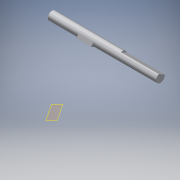
# Autodesk Inventor part: Shaft
Saved by Autodesk Inventor 2017 (Build 210142000, 142)
## iProperties
Created: 2018-02-26
Part Number: Shaft
Material: PAEK Plastic
Document SubType Name: Modeling
Designer: bradl
Density: 1.32 g/cm^3
Appearance: Smooth - White
Author: bradl
Autodesk Inventor part; units mm, degrees
ref_plane "YZ Plane" through (0, 0, 0) normal (1, 0, 0) x (0, 1, 0)
ref_plane "XZ Plane" through (0, 0, 0) normal (0, 1, 0) x (-1, 0, 0)
ref_plane "XY Plane" through (0, 0, 0) normal (0, 0, 1) x (1, 0, 0)
sketch "Sketch1" plane through (0, 0, 0) normal (1, 0, 0) x (0, 1, 0)
  circle A0 centre (0, 0) radius 1.4986
  dimension "d0" = 2.9972
  constraints: 1 centre point, 1 coincident
  measures "d0" diameter of A0
extrude "Extrusion1" add sketch "Sketch1" along normal blind 25.4
ref_plane "Work Plane1" through (7.81, -18.8269, 9.6237) normal (1, 0, 0) x (0, 0.4551504, 0.8904146)
sketch "Sketch2" plane through (7.81, -18.8269, 9.6237) normal (1, 0, 0) x (0, 0.4551504, 0.8904146)
  line L0 (0, -21.144) -> (-1.4986, -21.144) construction
  circle A0 centre (0, -21.144) radius 1.4986 construction
  line L1 (-1.4986, -21.144) -> (-1.4986, -19.6454)
  line L2 (-1.4986, -19.6454) -> (1.4986, -19.6454)
  line L3 (1.4986, -19.6454) -> (1.4986, -21.144)
  line L4 (-1.4986, -21.144) -> (1.4986, -21.144)
  constraints: 10 end point, 2 point on circle, 2 tangent, 1 collinear, 1 perpendicular, 1 vertical
extrude "Extrusion2" add sketch "Sketch2" along normal blind 5.08
sketch "Sketch3" plane through (25.4, 0, 0) normal (1, 0, 0) x (0, 0, -1)
  circle A0 centre (0, 0) radius 1.4986
  constraints: 1 centre point, 1 coincident
extrude "Extrusion3" add sketch "Sketch3" along normal blind 1.27
sketch "Sketch4" plane through (26.67, 0, 0) normal (1, 0, 0) x (0, 0, -1)
  line L0 (-0.5404, 1.3993) -> (1.4507, 0.3815)
  arc A0 (-10.1641, -17.4276) -> (-8.173, -18.4454) centre (-9.6237, -18.8269) ccw
  line L1 (-10.1641, -17.4276) -> (-8.173, -18.4454) projected
  line L2 (-2.0165, -0.6523) -> (-0.6821, -1.3344) projected
  arc A1 (1.4507, 0.3815) -> (-0.5404, 1.3993) centre (0, 0) ccw
  constraints: 4 point on circle, 2 centre point, 2 end point, 1 parallel, 4 other
extrude "Extrusion4" cut sketch "Sketch4" against normal blind 5.08 contours A1 L0
sketch "Sketch5" plane through (26.67, 0, 0) normal (1, 0, 0) x (0, 0, -1)
  line L0 (1.449, 0.3824) -> (-0.5387, 1.3984) projected
  line L1 (1.449, 0.3824) -> (-0.5387, 1.3984) projected
  arc A0 (-0.5387, 1.3984) -> (1.449, 0.3824) centre (0, 0) ccw projected
extrude "Extrusion5" add sketch "Sketch5" along normal blind 7.9375
sketch "Sketch6" plane through (0, 0, 0) normal (-1, 0, 0) x (0, 0, 1)
  arc A0 (-1.3344, -0.6821) -> (0.6821, -1.3344) centre (0, 0) ccw projected
  circle A1 centre (0, 0) radius 1.4986
  constraints: 1 coincident, 3 other
extrude "Extrusion6" add sketch "Sketch6" along normal blind 2.54
body "Solid1"
